Autodesk Fusion 360 part; units mm, degrees
(part 3 of 3)
sketch "草图1" plane through (0, 0, 0) normal (0, 0, 1) x (1, 0, 0)
  line L0 (8.5, 10) -> (-8.5, 10)
  line L1 (-10, 8.5) -> (-10, -8.5)
  line L2 (-8.5, -10) -> (8.5, -10)
  line L3 (10, -8.5) -> (10, 8.5)
  line L4 (10, 10) -> (-10, -10) construction
  line L5 (-10, 10) -> (10, -10) construction
  line L6 (12.5, 15) -> (-12.5, 15)
  line L7 (-12.5, 15) -> (-12.5, -18)
  line L8 (-12.5, -18) -> (12.5, -18)
  line L9 (12.5, -18) -> (12.5, 15)
  line L10 (12.5, 15) -> (-12.5, -18) construction
  line L11 (-12.5, 15) -> (12.5, -18) construction
  arc A0 (10, 8.5) -> (8.5, 10) centre (8.5, 8.5) ccw
  arc A1 (8.5, -10) -> (10, -8.5) centre (8.5, -8.5) ccw
  arc A2 (-10, -8.5) -> (-8.5, -10) centre (-8.5, -8.5) ccw
  arc A3 (-8.5, 10) -> (-10, 8.5) centre (-8.5, 8.5) ccw
  line L12 (0, -1.5) -> (0, 0) construction
  point P0 (0, -1.5)
  dimension "d2" = 20
  dimension "d3" = 25
  dimension "d4" = 1.5
  dimension "d138" = 20
  dimension "d139" = 20
  dimension "d140" = 33
  dimension "d141" = 15
  constraint horizontal L0
  constraint perpendicular L0 L1
  constraint parallel L0 L2
  constraint parallel L1 L3
  constraint coincident L4 L12.end
  constraint coincident L5 L12.end
  constraint coincident L12.end origin
  constraint horizontal L6
  constraint perpendicular L6 L7
  constraint parallel L6 L8
  constraint parallel L7 L9
  constraint coincident L4.start L0
  constraint coincident L4.start L3
  constraint tangent L0 A0
  constraint tangent L3 A0
  constraint coincident L5.end L3
  constraint coincident L5.end L2
  constraint tangent L3 A1
  constraint tangent L2 A1
  constraint equal A0 A1
  constraint coincident L4.end L2
  constraint coincident L4.end L1
  constraint tangent L2 A2
  constraint tangent L1 A2
  constraint equal A0 A2
  constraint coincident L5.start L1
  constraint coincident L5.start L0
  constraint tangent L1 A3
  constraint tangent L0 A3
  constraint equal A0 A3
  constraint coincident L9.end L6
  constraint coincident L6.start L9
  constraint coincident L8.end L9
  constraint coincident L9.start L8
  constraint coincident L7.end L8
  constraint coincident L8.start L7
  constraint coincident L6.end L7
  constraint coincident L7.start L6
  constraint midpoint L11 P0
  constraint coincident P0 L12.start
  constraint vertical L12
  constraint coincident L8.end L9.start
  constraint coincident L7.end L8.start
  constraint coincident L6.end L7.start
  constraint coincident L6.start L9.end
  measures "d2" distance of L4.start L5.start
  measures "d3" distance of L6.start L6.end
  measures "d4" radius of A0
  measures "d138" distance of L0 L2
  measures "d139" distance of L1 L3
  measures "d140" distance of L6 L8
  measures "d141" distance of L12.end L6
extrude "拉伸1" add sketch "草图1" along normal blind 20
sketch "草图17" plane through (0, 0, 0) normal (1, 0, 0) x (0, 1, 0)
  line L0 (0, 80.0802) -> (0, -28.3534) construction
  circle A0 centre (0, 5) radius 2
  dimension "d230" = 4
  dimension "d231" = 5
  constraint vertical L0
  constraint coincident L0 origin
  constraint coincident L0 A0.centre
  measures "d230" diameter of A0
  measures "d231" distance of origin A0.centre
extrude "拉伸16" cut sketch "草图17" along normal mid plane 40
sketch "草图18" plane through (0, 0, 0) normal (0, 1, 0) x (1, 0, 0)
  circle A0 centre (0, -11) radius 1.5
  circle A1 centre (9, -3) radius 1.5
  line L0 (0, -22) -> (0, 9.9016) construction
  line L1 (-12.5, 0) -> (12.5, 0)
  circle A2 centre (-9, -3) radius 1.5
  dimension "d239" = 3
  dimension "d240" = 3
  dimension "d241" = 3
  dimension "d242" = 11
  dimension "d243" = 9
  constraint vertical L0
  constraint coincident origin L0
  constraint coincident A0.centre L0
  constraint symmetric A1 L0 A2
  measures "d239" diameter of A0
  measures "d240" diameter of A1
  measures "d241" distance of A1.centre L1
  measures "d242" distance of A0.centre L1
  measures "d243" distance of A1.centre L0
sketch "草图20" plane through (0, 15, 0) normal (0, 1, 0) x (-1, 0, 0)
  line L0 (-12.5, 0) -> (12.5, 0)
  line L1 (12.5, 0) -> (12.5, 20)
  line L2 (12.5, 20) -> (-12.5, 20)
  line L3 (-12.5, 20) -> (-12.5, 0)
  circle A0 centre (9, 3) radius 1.5
  line L4 (12.5, 0) -> (-12.5, 0)
  circle A1 centre (0, 11) radius 1.5
  line L5 (0, 22) -> (0, -9.9016) construction
  circle A2 centre (-9, 3) radius 1.5
  point P0 (0, 0)
  dimension "d244" = 3
  dimension "d245" = 3
  dimension "d246" = 3
  dimension "d247" = 11
  dimension "d248" = 9
  constraint coincident P0 L5
  constraint coincident A1.centre L5
  constraint symmetric A0 L5 A2
  measures "d244" diameter of A1
  measures "d245" diameter of A2
  measures "d246" distance of A2.centre L4
  measures "d247" distance of A1.centre L4
  measures "d248" distance of A2.centre L5
sketch "草图21" plane through (0, -18, 0) normal (0, -1, 0) x (1, 0, 0)
  line L0 (-12.5, 0) -> (12.5, 0)
  line L1 (12.5, 0) -> (12.5, 20)
  line L2 (12.5, 20) -> (-12.5, 20)
  line L3 (-12.5, 20) -> (-12.5, 0)
  circle A0 centre (9, 3) radius 1.5
  line L4 (12.5, 0) -> (-12.5, 0)
  circle A1 centre (0, 11) radius 1.5
  line L5 (0, 22) -> (0, -9.9016) construction
  circle A2 centre (-9, 3) radius 1.5
  point P0 (0, 0)
  dimension "d249" = 3
  dimension "d250" = 3
  dimension "d251" = 3
  dimension "d252" = 11
  dimension "d253" = 9
  constraint coincident P0 L5
  constraint coincident A1.centre L5
  constraint symmetric A0 L5 A2
  measures "d249" diameter of A1
  measures "d250" diameter of A2
  measures "d251" distance of A2.centre L4
  measures "d252" distance of A1.centre L4
  measures "d253" distance of A2.centre L5
hole "孔4" at (0, 15, 11) at (-9, 15, 3) at (9, 15, 3) direction (0, -1, 0) diameter 2.529 depth 4 tip angle 118
thread "螺纹3" "ISO Metric profile 3.0 M3x0.5 6H" major diameter 3.086 minor diameter 2.529 pitch 0.5 angle 60 resizes the face on face at (-8.8741, 12.3333, 4.2582) on face at (0.1259, 12.3333, 12.2582) on face at (9.1259, 12.3333, 4.2582)
hole "孔5" at (0, -18, 11) at (9, -18, 3) at (-9, -18, 3) direction (0, 1, 0) diameter 2.529 depth 5 tip angle 118
thread "螺纹4" "ISO Metric profile 3.0 M3x0.5 6H" major diameter 3.086 minor diameter 2.529 pitch 0.5 angle 60 resizes the face on face at (0.063, -16.3333, 9.7371) on face at (9.063, -16.3333, 1.7371) on face at (-8.937, -16.3333, 1.7371)

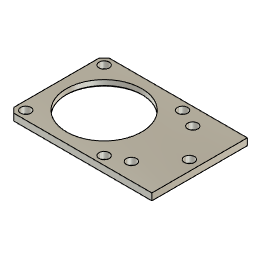
design "28电机输出固定"
Autodesk Fusion 360 part; units mm, degrees
sketch "草图1" plane through (0, 0, 0) normal (0, 0, 1) x (1, 0, 0)
  circle A0 centre (0, 0) radius 11.025
  line L0 (12.5, 14) -> (-12.5, 14)
  line L1 (-14, 12.5) -> (-14, -12.5)
  line L2 (-12.5, -14) -> (12.5, -14)
  line L3 (14, -12.5) -> (14, 12.5)
  line L4 (14, 14) -> (-14, -14) construction
  line L5 (-14, 14) -> (14, -14) construction
  circle A1 centre (11.5, -11.5) radius 1.5
  circle A2 centre (11.5, 11.5) radius 1.5
  circle A3 centre (-11.5, 11.5) radius 1.5
  circle A4 centre (-11.5, -11.5) radius 1.5
  line L6 (-12.5, 14) -> (-14, 12.5)
  line L7 (-14, -12.5) -> (-12.5, -14)
  line L8 (12.5, 14) -> (14, 12.5)
  line L9 (14, -12.5) -> (12.5, -14)
  line L10 (28, 14) -> (28, -14)
  line L11 (14, -18) -> (14, 12.5)
  line L12 (12.5, 14) -> (28, 14)
  line L13 (28, -14) -> (12.5, -14)
  circle A5 centre (25, 0) radius 1.5
  circle A6 centre (17, -9) radius 1.5
  line L14 (79.2108, 0) -> (-40, 0) construction
  circle A7 centre (17, 9) radius 1.5
  dimension "d1" = 22.05
  dimension "d2" = 28
  dimension "d3" = 28
  dimension "d4" = 11.5
  dimension "d5" = 3
  dimension "d7" = 360
  dimension "d8" = 1.5
  dimension "d9" = 1.5
  dimension "d10" = 1.5
  dimension "d11" = 1.5
  dimension "d12" = 1.5
  dimension "d13" = 1.5
  dimension "d14" = 1.5
  dimension "d15" = 1.5
  dimension "d17" = 14
  dimension "d20" = 3
  dimension "d21" = 3
  dimension "d24" = 9
  dimension "d26" = 11
  dimension "d27" = 3
  constraint coincident A0.centre origin
  constraint horizontal L0
  constraint perpendicular L0 L1
  constraint parallel L0 L2
  constraint parallel L1 L3
  constraint coincident L4 A0.centre
  constraint coincident L5 A0.centre
  constraint coincident L5 A1.centre
  constraint coincident L5.start L0
  constraint coincident L5.start L1
  constraint coincident L4.end L1
  constraint coincident L4.end L2
  constraint coincident L4.start L0
  constraint coincident L4.start L3
  constraint coincident L5.end L3
  constraint coincident L5.end L2
  constraint vertical L10
  constraint vertical L11
  constraint horizontal L12
  constraint horizontal L13
  constraint horizontal L14
  constraint coincident A0.centre L14
  constraint coincident A5.centre L14
  constraint symmetric A6 L14 A7
  measures "d1" diameter of A0
  measures "d2" distance of L4.start L5.start
  measures "d3" distance of L4.start L5.end
  measures "d4" horizontal distance of A0.centre A1.centre
  measures "d5" diameter of A1
  measures "d8" distance of L5.start L0.end
  measures "d9" distance of L5.start L1.start
  measures "d10" distance of L4.end L1.end
  measures "d11" distance of L4.end L2.start
  measures "d12" distance of L4.start L0.start
  measures "d13" distance of L4.start L3.end
  measures "d14" distance of L5.end L3.start
  measures "d15" distance of L5.end L2.end
  measures "d17" distance of L10 L11
  measures "d20" diameter of A6
  measures "d21" diameter of A5
  measures "d24" distance of A6.centre L14
  measures "d26" distance of L11 A5.centre
  measures "d27" distance of L11 A6.centre
extrude "拉伸1" add sketch "草图1" along normal blind 2
chamfer "倒角1" distance 0.5 angle 45 1 edges at (-10.2789, 3.9868, 0)
equation "d9 = d8"
equation "d11 = d10"
equation "d13 = d12"
equation "d15 = d14"
